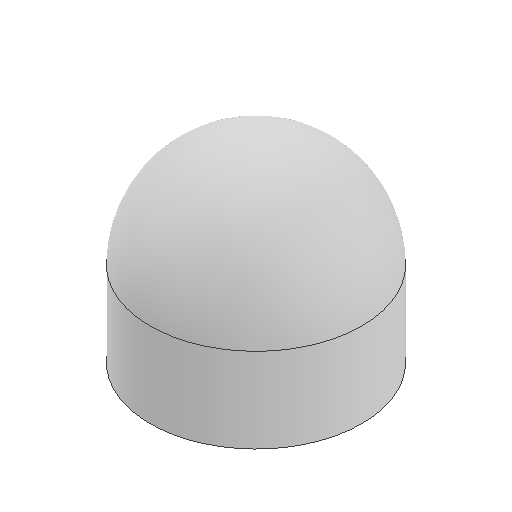
# Autodesk Inventor part: TAPA
Saved by Autodesk Inventor 2025.2 (Build 292293000, 293)
## iProperties
Created: 2025-09-12
Part Number: TAPA
Material: Generic
Document SubType Name: Modeling
Designer: Compa
Density: 1 g/cm^3
Appearance: Default
Author: Compa
Autodesk Inventor part; units mm, degrees
ref_plane "YZ Plane" through (0, 0, 0) normal (1, 0, 0) x (0, 1, 0)
ref_plane "XZ Plane" through (0, 0, 0) normal (0, 1, 0) x (-1, 0, 0)
ref_plane "XY Plane" through (0, 0, 0) normal (0, 0, 1) x (1, 0, 0)
sketch "Sketch6" plane through (0, 0, 0) normal (0, 0, 1) x (1, 0, 0)
  line L0 (0, 0) -> (11.5, 0)
  line L1 (11.5, 0) -> (11.5, -10)
  line L2 (11.5, -10) -> (12.5, -10)
  line L3 (12.5, -10) -> (12.5, 0)
  arc A0 (12.5, 0) -> (0, 12.5) centre (0, 0) ccw
  line L4 (0, 0) -> (0, 12.5) construction
  line L5 (0, 0) -> (12.5, 0) construction
  line L6 (0, 12.5) -> (0, 0)
  dimension "d51" = 11.5
  dimension "d52" = 10
  dimension "d53" = 1
  dimension "d54" = 90
  constraints: 14 end point, 2 horizontal, 2 perpendicular, 2 point on circle, 1 centre point, 1 coincident, 1 vertical
  measures "d51" distance of L0.start L0.end
  measures "d52" distance of L0.end L1.end
  measures "d53" distance of L1.end L2.end
  measures "d54" angle of L5 L4
revolve "Revolution4" add sketch "Sketch6" angle 360 about axis through (0, 12.5, 0) along (0, -1, 0)
thread "Thread4" size "M22x2" class "6H" standard "ANSI Metric M Profile" full length
sketch "Sketch8" plane through (0, -10, 0) normal (-1, 0, 0) x (0, 0, 1)
  line L0 (11.5, 0) -> (11.5, 10)
  line L1 (11.5, 10) -> (10.0171, 10)
  line L2 (10.0171, 10) -> (10.0171, 0)
  line L3 (10.0171, 0) -> (11.5, 0)
  line L4 (0, -7.1171) -> (0, 27.4362) projected
  constraints: 8 end point
revolve "Revolution5" add sketch "Sketch8" angle 360 about axis through (0, -10, 0) along (0, 1, 0) separate body
sketch "Sketch7" plane through (0, -10, 11.5) normal (1, 0, 0) x (0, 1, 0)
  line L0 (-1.1668, -0.1013) -> (-1.0001, -0.1013) construction
  line L1 (0.1666, -1.382) -> (-0.0001, -1.7021) construction
  line L2 (-2.0001, -1.7021) -> (-2.1668, -1.382) construction
  line L3 (-0.8334, -0.1013) -> (-1.0001, 0.2189) construction
  line L4 (-1.0001, 0.2189) -> (-1.1668, -0.1013) construction
  line L5 (-2.0001, -1.7021) -> (-1.8334, -1.382) construction
  line L6 (-0.8334, -0.1013) -> (-0.1668, -1.382)
  line L7 (-2.1668, -1.382) -> (-1.8334, -1.382) construction
  arc A0 (-2.1668, -1.382) -> (-2.0001, -1.4831) centre (-2.0001, -1.2952) ccw construction
  line L8 (0.1666, -1.382) -> (-0.1668, -1.382) construction
  line L9 (-2.0001, -1.7021) -> (-2.0001, -1.382) construction
  line L10 (-0.0001, -1.7021) -> (-0.0001, -1.382) construction
  line L11 (-1.0001, 0.2189) -> (-1.0001, -0.0002) construction
  line L12 (-2.0001, -1.4831) -> (-0.0001, -1.4831)
  arc A1 (-2.0001, -1.4831) -> (-1.8334, -1.382) centre (-2.0001, -1.2952) ccw
  line L13 (-0.1668, -1.382) -> (-0.0001, -1.7021) construction
  line L14 (-1.8334, -1.382) -> (-1.1668, -0.1013)
  line L15 (-0.0001, -0.0002) -> (-0.0001, 0.0177)
  line L16 (-0.0001, 0.0177) -> (-0.0001, -0.0002)
  line L17 (-0.0001, -0.0002) -> (0.0334, -0.0002)
  arc A2 (-0.1668, -1.382) -> (-0.0001, -1.4831) centre (-0.0001, -1.2952) ccw
  arc A3 (-0.0001, -1.4831) -> (0.1666, -1.382) centre (-0.0001, -1.2952) ccw construction
  arc A4 (-1.0001, -0.0002) -> (-1.1668, -0.1013) centre (-1.0001, -0.1881) ccw
  arc A5 (-0.8334, -0.1013) -> (-1.0001, -0.0002) centre (-1.0001, -0.1881) ccw
  line L18 (-1.0001, -0.0002) -> (-1.0001, -0.1013) construction
  line L19 (-1.0001, -0.1013) -> (-0.8334, -0.1013) construction
  dimension "d60" = 55
  dimension "d61" = 0.3202
  dimension "d62" = 0.3202
  dimension "Sketch7_ThreadOffset" = 0
  dimension "Sketch7_MajorRadius" = 1.4829
  dimension "d65" = 2
  dimension "Sketch7_MinorRadius" = 0
  constraints: 40 end point, 12 point on circle, 10 parallel, 8 tangent, 6 centre point, 6 collinear, 2 midpoint, 2 point on line, 1 horizontal, 1 perpendicular, 3 other
  measures "d60" angle of L6 L14
  measures "d61" distance of L3.end L0.end
  measures "d62" distance of L1.end L10.end
  measures "Sketch7_ThreadOffset" distance between parallel lines of L15 L10
  measures "Sketch7_MajorRadius" distance from line of L12 L15.start
  measures "d65" distance from line of L1.end L9
  measures "Sketch7_MinorRadius" distance edge to line of A5 L17
coil "Coil3" sketch "Sketch7" operation cut axis through (0, -10, 0) along (0, 1, 0) pitch 2.002 turns 6.993007 hand right bodies 2
equation "\"d60\" = d67"
equation "\"d61\" = 0.160083 * Sketch7_Pitch"
equation "\"d62\" = 0.160083 * Sketch7_Pitch"
equation "\"d65\" = Sketch7_Pitch"
equation "\"d16\" = 55deg"
equation "\"Sketch2_Pitch\" = 1"
equation "\"d36\" = 55deg"
equation "\"Sketch4_Pitch\" = 2.5"
equation "\"d67\" = 55deg"
equation "\"Sketch7_Pitch\" = 2"
body "Solid4"
body "Solid5"
